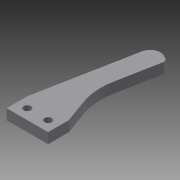
# Autodesk Inventor part: gripper
Saved by Autodesk Inventor 2015 (Build 190159000, 159)
## iProperties
Created: 2016-10-14
Part Number: gripper
Material: Generic
Document SubType Name: Modeling
Designer: Bardo91
Density: 1 g/cm^3
Appearance: Default
Author: Bardo91
Autodesk Inventor part; units mm, degrees
ref_plane "YZ Plane" through (0, 0, 0) normal (1, 0, 0) x (0, 1, 0)
ref_plane "XZ Plane" through (0, 0, 0) normal (0, 1, 0) x (-1, 0, 0)
ref_plane "XY Plane" through (0, 0, 0) normal (0, 0, 1) x (1, 0, 0)
sketch "Sketch1" plane through (0, 0, 0) normal (0, 0, 1) x (1, 0, 0)
  line L0 (0, 0) -> (5, 0)
  line L1 (5, 0) -> (-5, 0)
  circle A0 centre (-5, 0) radius 1.75
  circle A1 centre (5, 0) radius 1.75
  line L2 (0, 0) -> (0, -5)
  line L3 (0, -5) -> (10, -5)
  line L4 (10, -5) -> (10, 5)
  line L5 (0, -5) -> (-10, -5)
  line L6 (-10, -5) -> (-10, 5)
  line L7 (10, 5) -> (5.9879, 16.023)
  line L8 (10, 5) -> (21.7305, 5) construction
  line L9 (4.7122, 31.9163) -> (8.5293, 51.8848)
  line L10 (7.5896, 53.9779) -> (6.3368, 54.7253)
  line L11 (-1.1361, 51.3703) -> (-10, 5)
  arc A2 (4.7122, 31.9163) -> (5.9879, 16.023) centre (34.1787, 26.2837) ccw
  arc A3 (8.5293, 51.8848) -> (7.5896, 53.9779) centre (6.5649, 52.2603) ccw
  arc A4 (6.3368, 54.7253) -> (-1.1361, 51.3703) centre (3.775, 50.4315) ccw
  point P0 (3.1596, 23.7939)
  point P1 (8.7922, 53.2603)
  point P2 (0.2046, 58.384)
  dimension "d0" = 5
  dimension "d1" = 10
  dimension "d2" = 3.5
  dimension "d3" = 3.5
  dimension "d4" = 5
  dimension "d5" = 10
  dimension "d6" = 10
  dimension "d7" = 10
  dimension "d8" = 10
  dimension "d9" = 20
  dimension "d10" = 110
  dimension "d11" = 30
  dimension "d12" = 10
  dimension "d13" = 110
  dimension "d14" = 30
  dimension "d15" = 2
  dimension "d16" = 5
  constraints: 24 end point, 7 point on line, 6 point on circle, 6 tangent, 5 centre point, 3 horizontal, 3 perpendicular, 2 coincident, 1 equal length, 1 parallel, 1 vertical
  measures "d0" distance of L0.start L0.end
  measures "d1" distance of L0.end L1.end
  measures "d2" diameter of A0
  measures "d3" diameter of A1
  measures "d4" distance of L0.start L2.end
  measures "d5" distance of L2.end L3.end
  measures "d6" distance of L3.end L4.end
  measures "d7" distance of L2.end L5.end
  measures "d8" distance of L5.end L6.end
  measures "d9" distance of L4.end point (3.16, 23.794)
  measures "d10" angle of L8 L7
  measures "d11" distance of point (3.16, 23.794) point (8.792, 53.26)
  measures "d12" distance of point (8.792, 53.26) point (0.205, 58.384)
  measures "d13" angle of L10 L9
  measures "d14" radius of A2
  measures "d15" radius of A3
  measures "d16" radius of A4
extrude "Extrusion1" add sketch "Sketch1" along normal blind 5
body "Solid1"
